Autodesk Fusion 360 part; units mm, degrees
(part 2 of 3)
sketch "Sketch4" plane through (0, 0, 1.5) normal (0, 0, 1) x (-1, 0, 0) in component "Plate"
  line L0 (-48.7193, -101.035) -> (-62.72, -101.035)
  line L1 (-62.72, -101.035) -> (-62.72, -87.0356)
  line L2 (-62.72, -87.0356) -> (-48.7193, -87.0356)
  line L3 (-48.7193, -87.0356) -> (-48.7193, -101.035)
  line L4 (-24.62, -67.9856) -> (-10.6192, -67.9856)
  line L5 (-10.6192, -67.9856) -> (-10.6192, -81.9848)
  line L6 (-10.6192, -81.9848) -> (-24.62, -81.9848)
  line L7 (-24.62, -81.9848) -> (-24.62, -67.9856)
  line L8 (-81.77, -72.4598) -> (-81.77, -58.4606)
  line L9 (-81.77, -58.4606) -> (-77.0696, -58.4606)
  line L10 (-77.0696, -58.4606) -> (-77.0696, -56.9352)
  line L11 (-77.0696, -56.9352) -> (-80.2996, -56.9352)
  line L12 (-80.2996, -56.9352) -> (-80.2996, -55.2097)
  line L13 (-80.2996, -55.2097) -> (-81.219, -55.2097)
  line L14 (-81.219, -55.2097) -> (-81.219, -51.9105)
  line L15 (-81.219, -51.9105) -> (-80.2996, -51.9105)
  line L16 (-80.2996, -51.9105) -> (-80.2996, -50.1855)
  line L17 (-80.2996, -50.1855) -> (-77.0696, -50.1855)
  line L18 (-77.0696, -50.1855) -> (-77.0696, -49.36)
  line L19 (-77.0696, -49.36) -> (-74.2692, -49.36)
  line L20 (-74.2692, -49.36) -> (-74.2692, -50.1855)
  line L21 (-74.2692, -50.1855) -> (-67.9993, -50.1855)
  line L22 (-67.9993, -50.1855) -> (-67.9993, -51.9105)
  line L23 (-67.9993, -51.9105) -> (-67.0197, -51.9105)
  line L24 (-67.0197, -51.9105) -> (-67.0197, -55.2097)
  line L25 (-67.0197, -55.2097) -> (-67.9993, -55.2097)
  line L26 (-67.9993, -55.2097) -> (-67.9993, -56.9352)
  line L27 (-67.9993, -56.9352) -> (-72.4697, -56.9352)
  line L28 (-72.4697, -56.9352) -> (-72.4697, -58.4606)
  line L29 (-72.4697, -58.4606) -> (-67.7693, -58.4606)
  line L30 (-67.7693, -58.4606) -> (-67.7693, -72.4598)
  line L31 (-67.7693, -72.4598) -> (-72.4697, -72.4598)
  line L32 (-72.4697, -72.4598) -> (-72.4697, -73.9856)
  line L33 (-72.4697, -73.9856) -> (-67.9993, -73.9856)
  line L34 (-67.9993, -73.9856) -> (-67.9993, -75.7107)
  line L35 (-67.9993, -75.7107) -> (-67.0197, -75.7107)
  line L36 (-67.0197, -75.7107) -> (-67.0197, -79.0099)
  line L37 (-67.0197, -79.0099) -> (-67.9993, -79.0099)
  line L38 (-67.9993, -79.0099) -> (-67.9993, -80.735)
  line L39 (-67.9993, -80.735) -> (-74.2692, -80.735)
  line L40 (-74.2692, -80.735) -> (-74.2692, -81.5605)
  line L41 (-74.2692, -81.5605) -> (-77.0696, -81.5605)
  line L42 (-77.0696, -81.5605) -> (-77.0696, -80.735)
  line L43 (-77.0696, -80.735) -> (-80.2996, -80.735)
  line L44 (-80.2996, -80.735) -> (-80.2996, -79.0099)
  line L45 (-80.2996, -79.0099) -> (-81.219, -79.0099)
  line L46 (-81.219, -79.0099) -> (-81.219, -75.7107)
  line L47 (-81.219, -75.7107) -> (-80.2996, -75.7107)
  line L48 (-80.2996, -75.7107) -> (-80.2996, -73.9856)
  line L49 (-80.2996, -73.9856) -> (-77.0696, -73.9856)
  line L50 (-77.0696, -73.9856) -> (-77.0696, -72.4598)
  line L51 (-77.0696, -72.4598) -> (-81.77, -72.4598)
  line L52 (-24.62, -101.035) -> (-24.62, -87.0356)
  line L53 (-24.62, -87.0356) -> (-10.6192, -87.0356)
  line L54 (-10.6192, -87.0356) -> (-10.6192, -101.035)
  line L55 (-10.6192, -101.035) -> (-24.62, -101.035)
  line L56 (-31.4446, -129.035) -> (-60.9446, -129.035)
  line L57 (-60.9446, -129.035) -> (-60.9446, -114.035)
  line L58 (-60.9446, -114.035) -> (-31.4446, -114.035)
  line L59 (-31.4446, -114.035) -> (-31.4446, -129.035)
  line L60 (-81.77, -87.0356) -> (-67.7693, -87.0356)
  line L61 (-67.7693, -87.0356) -> (-67.7693, -101.035)
  line L62 (-67.7693, -101.035) -> (-81.77, -101.035)
  line L63 (-81.77, -101.035) -> (-81.77, -87.0356)
  line L64 (-62.72, -67.9856) -> (-48.7193, -67.9856)
  line L65 (-48.7193, -67.9856) -> (-48.7193, -81.9848)
  line L66 (-48.7193, -81.9848) -> (-62.72, -81.9848)
  line L67 (-62.72, -81.9848) -> (-62.72, -67.9856)
  line L68 (-29.6692, -67.9856) -> (-29.6692, -81.9848)
  line L69 (-29.6692, -81.9848) -> (-43.67, -81.9848)
  line L70 (-43.67, -81.9848) -> (-43.67, -67.9856)
  line L71 (-43.67, -67.9856) -> (-29.6692, -67.9856)
  line L72 (-29.6692, -48.9356) -> (-29.6692, -62.9348)
  line L73 (-29.6692, -62.9348) -> (-43.67, -62.9348)
  line L74 (-43.67, -62.9348) -> (-43.67, -48.9356)
  line L75 (-43.67, -48.9356) -> (-29.6692, -48.9356)
  line L76 (-67.9993, -12.0854) -> (-67.9993, -13.8107)
  line L77 (-67.9993, -13.8107) -> (-67.0197, -13.8107)
  line L78 (-67.0197, -13.8107) -> (-67.0197, -17.1097)
  line L79 (-67.0197, -17.1097) -> (-67.9993, -17.1097)
  line L80 (-67.9993, -17.1097) -> (-67.9993, -18.835)
  line L81 (-67.9993, -18.835) -> (-72.4697, -18.835)
  line L82 (-72.4697, -18.835) -> (-72.4697, -20.3605)
  line L83 (-72.4697, -20.3605) -> (-67.7693, -20.3605)
  line L84 (-67.7693, -20.3605) -> (-67.7693, -34.36)
  line L85 (-67.7693, -34.36) -> (-72.4697, -34.36)
  line L86 (-72.4697, -34.36) -> (-72.4697, -35.8856)
  line L87 (-72.4697, -35.8856) -> (-67.9993, -35.8856)
  line L88 (-67.9993, -35.8856) -> (-67.9993, -37.6107)
  line L89 (-67.9993, -37.6107) -> (-67.0197, -37.6107)
  line L90 (-67.0197, -37.6107) -> (-67.0197, -40.9099)
  line L91 (-67.0197, -40.9099) -> (-67.9993, -40.9099)
  line L92 (-67.9993, -40.9099) -> (-67.9993, -42.635)
  line L93 (-67.9993, -42.635) -> (-74.2692, -42.635)
  line L94 (-74.2692, -42.635) -> (-74.2692, -43.4605)
  line L95 (-74.2692, -43.4605) -> (-77.0696, -43.4605)
  line L96 (-77.0696, -43.4605) -> (-77.0696, -42.635)
  line L97 (-77.0696, -42.635) -> (-80.2996, -42.635)
  line L98 (-80.2996, -42.635) -> (-80.2996, -40.9099)
  line L99 (-80.2996, -40.9099) -> (-81.219, -40.9099)
  line L100 (-81.219, -40.9099) -> (-81.219, -37.6107)
  line L101 (-81.219, -37.6107) -> (-80.2996, -37.6107)
  line L102 (-80.2996, -37.6107) -> (-80.2996, -35.8856)
  line L103 (-80.2996, -35.8856) -> (-77.0696, -35.8856)
  line L104 (-77.0696, -35.8856) -> (-77.0696, -34.36)
  line L105 (-77.0696, -34.36) -> (-81.77, -34.36)
  line L106 (-81.77, -34.36) -> (-81.77, -20.3605)
  line L107 (-81.77, -20.3605) -> (-77.0696, -20.3605)
  line L108 (-77.0696, -20.3605) -> (-77.0696, -18.835)
  line L109 (-77.0696, -18.835) -> (-80.2996, -18.835)
  line L110 (-80.2996, -18.835) -> (-80.2996, -17.1097)
  line L111 (-80.2996, -17.1097) -> (-81.219, -17.1097)
  line L112 (-81.219, -17.1097) -> (-81.219, -13.8107)
  line L113 (-81.219, -13.8107) -> (-80.2996, -13.8107)
  line L114 (-80.2996, -13.8107) -> (-80.2996, -12.0854)
  line L115 (-80.2996, -12.0854) -> (-77.0696, -12.0854)
  line L116 (-77.0696, -12.0854) -> (-77.0696, -11.26)
  line L117 (-77.0696, -11.26) -> (-74.2692, -11.26)
  line L118 (-74.2692, -11.26) -> (-74.2692, -12.0854)
  line L119 (-74.2692, -12.0854) -> (-67.9993, -12.0854)
  line L120 (-29.6692, -29.8855) -> (-29.6692, -43.8849)
  line L121 (-29.6692, -43.8849) -> (-43.67, -43.8849)
  line L122 (-43.67, -43.8849) -> (-43.67, -29.8855)
  line L123 (-43.67, -29.8855) -> (-29.6692, -29.8855)
  line L124 (-48.7193, -62.9348) -> (-62.72, -62.9348)
  line L125 (-62.72, -62.9348) -> (-62.72, -48.9356)
  line L126 (-62.72, -48.9356) -> (-48.7193, -48.9356)
  line L127 (-48.7193, -48.9356) -> (-48.7193, -62.9348)
  line L128 (-24.62, -43.8849) -> (-24.62, -29.8855)
  line L129 (-24.62, -29.8855) -> (-10.6192, -29.8855)
  line L130 (-10.6192, -29.8855) -> (-10.6192, -43.8849)
  line L131 (-10.6192, -43.8849) -> (-24.62, -43.8849)
  line L132 (-48.7193, -10.8355) -> (-48.7193, -24.835)
  line L133 (-48.7193, -24.835) -> (-62.72, -24.835)
  line L134 (-62.72, -24.835) -> (-62.72, -10.8355)
  line L135 (-62.72, -10.8355) -> (-48.7193, -10.8355)
  line L136 (-37.3944, -23.3646) -> (-37.3944, -24.2852)
  line L137 (-37.3944, -24.2852) -> (-40.6936, -24.2852)
  line L138 (-40.6936, -24.2852) -> (-40.6936, -23.3646)
  line L139 (-40.6936, -23.3646) -> (-42.4187, -23.3646)
  line L140 (-42.4187, -23.3646) -> (-42.4187, -20.1345)
  line L141 (-42.4187, -20.1345) -> (-43.2442, -20.1345)
  line L142 (-43.2442, -20.1345) -> (-43.2442, -17.3357)
  line L143 (-43.2442, -17.3357) -> (-42.4187, -17.3357)
  line L144 (-42.4187, -17.3357) -> (-42.4187, -11.0657)
  line L145 (-42.4187, -11.0657) -> (-40.6936, -11.0657)
  line L146 (-40.6936, -11.0657) -> (-40.6936, -10.0858)
  line L147 (-40.6936, -10.0858) -> (-37.3944, -10.0858)
  line L148 (-37.3944, -10.0858) -> (-37.3944, -11.0657)
  line L149 (-37.3944, -11.0657) -> (-35.669, -11.0657)
  line L150 (-35.669, -11.0657) -> (-35.669, -15.5346)
  line L151 (-35.669, -15.5346) -> (-34.145, -15.5346)
  line L152 (-34.145, -15.5346) -> (-34.145, -10.8355)
  line L153 (-34.145, -10.8355) -> (-20.1442, -10.8355)
  line L154 (-20.1442, -10.8355) -> (-20.1442, -15.5346)
  line L155 (-20.1442, -15.5346) -> (-18.6201, -15.5346)
  line L156 (-18.6201, -15.5346) -> (-18.6201, -11.0657)
  line L157 (-18.6201, -11.0657) -> (-16.8934, -11.0657)
  line L158 (-16.8934, -11.0657) -> (-16.8934, -10.0858)
  line L159 (-16.8934, -10.0858) -> (-13.593, -10.0858)
  line L160 (-13.593, -10.0858) -> (-13.593, -11.0657)
  line L161 (-13.593, -11.0657) -> (-11.869, -11.0657)
  line L162 (-11.869, -11.0657) -> (-11.869, -17.3357)
  line L163 (-11.869, -17.3357) -> (-11.0436, -17.3357)
  line L164 (-11.0436, -17.3357) -> (-11.0436, -20.1345)
  line L165 (-11.0436, -20.1345) -> (-11.869, -20.1345)
  line L166 (-11.869, -20.1345) -> (-11.869, -23.3646)
  line L167 (-11.869, -23.3646) -> (-13.593, -23.3646)
  line L168 (-13.593, -23.3646) -> (-13.593, -24.2852)
  line L169 (-13.593, -24.2852) -> (-16.8934, -24.2852)
  line L170 (-16.8934, -24.2852) -> (-16.8934, -23.3646)
  line L171 (-16.8934, -23.3646) -> (-18.6201, -23.3646)
  line L172 (-18.6201, -23.3646) -> (-18.6201, -20.1345)
  line L173 (-18.6201, -20.1345) -> (-20.1442, -20.1345)
  line L174 (-20.1442, -20.1345) -> (-20.1442, -24.835)
  line L175 (-20.1442, -24.835) -> (-34.145, -24.835)
  line L176 (-34.145, -24.835) -> (-34.145, -20.1345)
  line L177 (-34.145, -20.1345) -> (-35.669, -20.1345)
  line L178 (-35.669, -20.1345) -> (-35.669, -23.3646)
  line L179 (-35.669, -23.3646) -> (-37.3944, -23.3646)
  line L180 (-62.72, -43.8849) -> (-62.72, -29.8855)
  line L181 (-62.72, -29.8855) -> (-48.7193, -29.8855)
  line L182 (-48.7193, -29.8855) -> (-48.7193, -43.8849)
  line L183 (-48.7193, -43.8849) -> (-62.72, -43.8849)
  line L184 (-43.67, -87.0356) -> (-29.6692, -87.0356)
  line L185 (-29.6692, -87.0356) -> (-29.6692, -101.035)
  line L186 (-29.6692, -101.035) -> (-43.67, -101.035)
  line L187 (-43.67, -101.035) -> (-43.67, -87.0356)
  line L188 (-24.62, -62.9348) -> (-24.62, -48.9356)
  line L189 (-24.62, -48.9356) -> (-10.6192, -48.9356)
  line L190 (-10.6192, -48.9356) -> (-10.6192, -62.9348)
  line L191 (-10.6192, -62.9348) -> (-24.62, -62.9348)
  arc A0 (-6.6192, -142.035) -> (-4.6192, -140.035) centre (-6.6192, -140.035) ccw
  line L192 (-4.6192, -140.035) -> (-4.6192, -6.8355)
  arc A1 (-4.6192, -6.8355) -> (-6.6192, -4.8355) centre (-6.6192, -6.8355) ccw
  line L193 (-6.6192, -4.8355) -> (-85.77, -4.8355)
  arc A2 (-85.77, -4.8355) -> (-87.77, -6.8355) centre (-85.77, -6.8355) ccw
  line L194 (-87.77, -6.8355) -> (-87.77, -140.035)
  arc A3 (-87.77, -140.035) -> (-85.77, -142.035) centre (-85.77, -140.035) ccw
  line L195 (-85.77, -142.035) -> (-6.6192, -142.035)
  line L196 (-31.4446, -129.035) -> (-60.9446, -129.035)
  line L197 (-31.4446, -114.035) -> (-31.4446, -129.035)
  line L198 (-60.9446, -114.035) -> (-31.4446, -114.035)
  line L199 (-60.9446, -129.035) -> (-60.9446, -114.035)
  line L200 (-10.6192, -114.5353) -> (-10.6192, -128.5347)
  line L201 (-10.6192, -128.5347) -> (-24.62, -128.5347)
  line L202 (-24.62, -128.5347) -> (-24.62, -114.5353)
  line L203 (-24.62, -114.5353) -> (-10.6192, -114.5353)
sketch "Sketch5" plane through (0, 0, 0) normal (0, 0, -1) x (1, 0, 0) in component "Plate"
  line L0 (62.72, -101.035) -> (48.7193, -101.035)
  line L1 (48.7193, -101.035) -> (48.7193, -87.0356)
  line L2 (48.7193, -87.0356) -> (62.72, -87.0356)
  line L3 (62.72, -87.0356) -> (62.72, -101.035)
  line L4 (10.6192, -67.9856) -> (24.62, -67.9856)
  line L5 (24.62, -67.9856) -> (24.62, -81.9848)
  line L6 (24.62, -81.9848) -> (10.6192, -81.9848)
  line L7 (10.6192, -81.9848) -> (10.6192, -67.9856)
  line L8 (81.77, -58.4606) -> (81.77, -72.4598)
  line L9 (81.77, -72.4598) -> (77.0696, -72.4598)
  line L10 (77.0696, -72.4598) -> (77.0696, -73.9856)
  line L11 (77.0696, -73.9856) -> (80.2996, -73.9856)
  line L12 (80.2996, -73.9856) -> (80.2996, -75.7107)
  line L13 (80.2996, -75.7107) -> (81.219, -75.7107)
  line L14 (81.219, -75.7107) -> (81.219, -79.0099)
  line L15 (81.219, -79.0099) -> (80.2996, -79.0099)
  line L16 (80.2996, -79.0099) -> (80.2996, -80.735)
  line L17 (80.2996, -80.735) -> (77.0696, -80.735)
  line L18 (77.0696, -80.735) -> (77.0696, -81.5605)
  line L19 (77.0696, -81.5605) -> (74.2692, -81.5605)
  line L20 (74.2692, -81.5605) -> (74.2692, -80.735)
  line L21 (74.2692, -80.735) -> (67.9993, -80.735)
  line L22 (67.9993, -80.735) -> (67.9993, -79.0099)
  line L23 (67.9993, -79.0099) -> (67.0197, -79.0099)
  line L24 (67.0197, -79.0099) -> (67.0197, -75.7107)
  line L25 (67.0197, -75.7107) -> (67.9993, -75.7107)
  line L26 (67.9993, -75.7107) -> (67.9993, -73.9856)
  line L27 (67.9993, -73.9856) -> (72.4697, -73.9856)
  line L28 (72.4697, -73.9856) -> (72.4697, -72.4598)
  line L29 (72.4697, -72.4598) -> (67.7693, -72.4598)
  line L30 (67.7693, -72.4598) -> (67.7693, -58.4606)
  line L31 (67.7693, -58.4606) -> (72.4697, -58.4606)
  line L32 (72.4697, -58.4606) -> (72.4697, -56.9352)
  line L33 (72.4697, -56.9352) -> (67.9993, -56.9352)
  line L34 (67.9993, -56.9352) -> (67.9993, -55.2097)
  line L35 (67.9993, -55.2097) -> (67.0197, -55.2097)
  line L36 (67.0197, -55.2097) -> (67.0197, -51.9105)
  line L37 (67.0197, -51.9105) -> (67.9993, -51.9105)
  line L38 (67.9993, -51.9105) -> (67.9993, -50.1855)
  line L39 (67.9993, -50.1855) -> (74.2692, -50.1855)
  line L40 (74.2692, -50.1855) -> (74.2692, -49.36)
  line L41 (74.2692, -49.36) -> (77.0696, -49.36)
  line L42 (77.0696, -49.36) -> (77.0696, -50.1855)
  line L43 (77.0696, -50.1855) -> (80.2996, -50.1855)
  line L44 (80.2996, -50.1855) -> (80.2996, -51.9105)
  line L45 (80.2996, -51.9105) -> (81.219, -51.9105)
  line L46 (81.219, -51.9105) -> (81.219, -55.2097)
  line L47 (81.219, -55.2097) -> (80.2996, -55.2097)
  line L48 (80.2996, -55.2097) -> (80.2996, -56.9352)
  line L49 (80.2996, -56.9352) -> (77.0696, -56.9352)
  line L50 (77.0696, -56.9352) -> (77.0696, -58.4606)
  line L51 (77.0696, -58.4606) -> (81.77, -58.4606)
  line L52 (24.62, -87.0356) -> (24.62, -101.035)
  line L53 (24.62, -101.035) -> (10.6192, -101.035)
  line L54 (10.6192, -101.035) -> (10.6192, -87.0356)
  line L55 (10.6192, -87.0356) -> (24.62, -87.0356)
  line L56 (60.9446, -129.035) -> (31.4446, -129.035)
  line L57 (31.4446, -129.035) -> (31.4446, -114.035)
  line L58 (31.4446, -114.035) -> (60.9446, -114.035)
  line L59 (60.9446, -114.035) -> (60.9446, -129.035)
  line L60 (67.7693, -87.0356) -> (81.77, -87.0356)
  line L61 (81.77, -87.0356) -> (81.77, -101.035)
  line L62 (81.77, -101.035) -> (67.7693, -101.035)
  line L63 (67.7693, -101.035) -> (67.7693, -87.0356)
  line L64 (48.7193, -67.9856) -> (62.72, -67.9856)
  line L65 (62.72, -67.9856) -> (62.72, -81.9848)
  line L66 (62.72, -81.9848) -> (48.7193, -81.9848)
  line L67 (48.7193, -81.9848) -> (48.7193, -67.9856)
  line L68 (29.6692, -81.9848) -> (29.6692, -67.9856)
  line L69 (29.6692, -67.9856) -> (43.67, -67.9856)
  line L70 (43.67, -67.9856) -> (43.67, -81.9848)
  line L71 (43.67, -81.9848) -> (29.6692, -81.9848)
  line L72 (29.6692, -62.9348) -> (29.6692, -48.9356)
  line L73 (29.6692, -48.9356) -> (43.67, -48.9356)
  line L74 (43.67, -48.9356) -> (43.67, -62.9348)
  line L75 (43.67, -62.9348) -> (29.6692, -62.9348)
  line L76 (67.9993, -13.8107) -> (67.9993, -12.0854)
  line L77 (67.9993, -12.0854) -> (74.2692, -12.0854)
  line L78 (74.2692, -12.0854) -> (74.2692, -11.26)
  line L79 (74.2692, -11.26) -> (77.0696, -11.26)
  line L80 (77.0696, -11.26) -> (77.0696, -12.0854)
  line L81 (77.0696, -12.0854) -> (80.2996, -12.0854)
  line L82 (80.2996, -12.0854) -> (80.2996, -13.8107)
  line L83 (80.2996, -13.8107) -> (81.219, -13.8107)
  line L84 (81.219, -13.8107) -> (81.219, -17.1097)
  line L85 (81.219, -17.1097) -> (80.2996, -17.1097)
  line L86 (80.2996, -17.1097) -> (80.2996, -18.835)
  line L87 (80.2996, -18.835) -> (77.0696, -18.835)
  line L88 (77.0696, -18.835) -> (77.0696, -20.3605)
  line L89 (77.0696, -20.3605) -> (81.77, -20.3605)
  line L90 (81.77, -20.3605) -> (81.77, -34.36)
  line L91 (81.77, -34.36) -> (77.0696, -34.36)
  line L92 (77.0696, -34.36) -> (77.0696, -35.8856)
  line L93 (77.0696, -35.8856) -> (80.2996, -35.8856)
  line L94 (80.2996, -35.8856) -> (80.2996, -37.6107)
  line L95 (80.2996, -37.6107) -> (81.219, -37.6107)
  line L96 (81.219, -37.6107) -> (81.219, -40.9099)
  line L97 (81.219, -40.9099) -> (80.2996, -40.9099)
  line L98 (80.2996, -40.9099) -> (80.2996, -42.635)
  line L99 (80.2996, -42.635) -> (77.0696, -42.635)
  line L100 (77.0696, -42.635) -> (77.0696, -43.4605)
  line L101 (77.0696, -43.4605) -> (74.2692, -43.4605)
  line L102 (74.2692, -43.4605) -> (74.2692, -42.635)
  line L103 (74.2692, -42.635) -> (67.9993, -42.635)
  line L104 (67.9993, -42.635) -> (67.9993, -40.9099)
  line L105 (67.9993, -40.9099) -> (67.0197, -40.9099)
  line L106 (67.0197, -40.9099) -> (67.0197, -37.6107)
  line L107 (67.0197, -37.6107) -> (67.9993, -37.6107)
  line L108 (67.9993, -37.6107) -> (67.9993, -35.8856)
  line L109 (67.9993, -35.8856) -> (72.4697, -35.8856)
  line L110 (72.4697, -35.8856) -> (72.4697, -34.36)
  line L111 (72.4697, -34.36) -> (67.7693, -34.36)
  line L112 (67.7693, -34.36) -> (67.7693, -20.3605)
  line L113 (67.7693, -20.3605) -> (72.4697, -20.3605)
  line L114 (72.4697, -20.3605) -> (72.4697, -18.835)
  line L115 (72.4697, -18.835) -> (67.9993, -18.835)
  line L116 (67.9993, -18.835) -> (67.9993, -17.1097)
  line L117 (67.9993, -17.1097) -> (67.0197, -17.1097)
  line L118 (67.0197, -17.1097) -> (67.0197, -13.8107)
  line L119 (67.0197, -13.8107) -> (67.9993, -13.8107)
  line L120 (29.6692, -43.8849) -> (29.6692, -29.8855)
  line L121 (29.6692, -29.8855) -> (43.67, -29.8855)
  line L122 (43.67, -29.8855) -> (43.67, -43.8849)
  line L123 (43.67, -43.8849) -> (29.6692, -43.8849)
  line L124 (62.72, -62.9348) -> (48.7193, -62.9348)
  line L125 (48.7193, -62.9348) -> (48.7193, -48.9356)
  line L126 (48.7193, -48.9356) -> (62.72, -48.9356)
  line L127 (62.72, -48.9356) -> (62.72, -62.9348)
  line L128 (24.62, -29.8855) -> (24.62, -43.8849)
  line L129 (24.62, -43.8849) -> (10.6192, -43.8849)
  line L130 (10.6192, -43.8849) -> (10.6192, -29.8855)
  line L131 (10.6192, -29.8855) -> (24.62, -29.8855)
  line L132 (48.7193, -24.835) -> (48.7193, -10.8355)
  line L133 (48.7193, -10.8355) -> (62.72, -10.8355)
  line L134 (62.72, -10.8355) -> (62.72, -24.835)
  line L135 (62.72, -24.835) -> (48.7193, -24.835)
  line L136 (37.3944, -24.2852) -> (37.3944, -23.3646)
  line L137 (37.3944, -23.3646) -> (35.669, -23.3646)
  line L138 (35.669, -23.3646) -> (35.669, -20.1345)
  line L139 (35.669, -20.1345) -> (34.145, -20.1345)
  line L140 (34.145, -20.1345) -> (34.145, -24.835)
  line L141 (34.145, -24.835) -> (20.1442, -24.835)
  line L142 (20.1442, -24.835) -> (20.1442, -20.1345)
  line L143 (20.1442, -20.1345) -> (18.6201, -20.1345)
  line L144 (18.6201, -20.1345) -> (18.6201, -23.3646)
  line L145 (18.6201, -23.3646) -> (16.8934, -23.3646)
  line L146 (16.8934, -23.3646) -> (16.8934, -24.2852)
  line L147 (16.8934, -24.2852) -> (13.593, -24.2852)
  line L148 (13.593, -24.2852) -> (13.593, -23.3646)
  line L149 (13.593, -23.3646) -> (11.869, -23.3646)
  line L150 (11.869, -23.3646) -> (11.869, -20.1345)
  line L151 (11.869, -20.1345) -> (11.0436, -20.1345)
  line L152 (11.0436, -20.1345) -> (11.0436, -17.3357)
  line L153 (11.0436, -17.3357) -> (11.869, -17.3357)
  line L154 (11.869, -17.3357) -> (11.869, -11.0657)
  line L155 (11.869, -11.0657) -> (13.593, -11.0657)
  line L156 (13.593, -11.0657) -> (13.593, -10.0858)
  line L157 (13.593, -10.0858) -> (16.8934, -10.0858)
  line L158 (16.8934, -10.0858) -> (16.8934, -11.0657)
  line L159 (16.8934, -11.0657) -> (18.6201, -11.0657)
  line L160 (18.6201, -11.0657) -> (18.6201, -15.5346)
  line L161 (18.6201, -15.5346) -> (20.1442, -15.5346)
  line L162 (20.1442, -15.5346) -> (20.1442, -10.8355)
  line L163 (20.1442, -10.8355) -> (34.145, -10.8355)
  line L164 (34.145, -10.8355) -> (34.145, -15.5346)
  line L165 (34.145, -15.5346) -> (35.669, -15.5346)
  line L166 (35.669, -15.5346) -> (35.669, -11.0657)
  line L167 (35.669, -11.0657) -> (37.3944, -11.0657)
  line L168 (37.3944, -11.0657) -> (37.3944, -10.0858)
  line L169 (37.3944, -10.0858) -> (40.6936, -10.0858)
  line L170 (40.6936, -10.0858) -> (40.6936, -11.0657)
  line L171 (40.6936, -11.0657) -> (42.4187, -11.0657)
  line L172 (42.4187, -11.0657) -> (42.4187, -17.3357)
  line L173 (42.4187, -17.3357) -> (43.2442, -17.3357)
  line L174 (43.2442, -17.3357) -> (43.2442, -20.1345)
  line L175 (43.2442, -20.1345) -> (42.4187, -20.1345)
  line L176 (42.4187, -20.1345) -> (42.4187, -23.3646)
  line L177 (42.4187, -23.3646) -> (40.6936, -23.3646)
  line L178 (40.6936, -23.3646) -> (40.6936, -24.2852)
  line L179 (40.6936, -24.2852) -> (37.3944, -24.2852)
  line L180 (62.72, -29.8855) -> (62.72, -43.8849)
  line L181 (62.72, -43.8849) -> (48.7193, -43.8849)
  line L182 (48.7193, -43.8849) -> (48.7193, -29.8855)
  line L183 (48.7193, -29.8855) -> (62.72, -29.8855)
  line L184 (29.6692, -87.0356) -> (43.67, -87.0356)
  line L185 (43.67, -87.0356) -> (43.67, -101.035)
  line L186 (43.67, -101.035) -> (29.6692, -101.035)
  line L187 (29.6692, -101.035) -> (29.6692, -87.0356)
  line L188 (24.62, -48.9356) -> (24.62, -62.9348)
  line L189 (24.62, -62.9348) -> (10.6192, -62.9348)
  line L190 (10.6192, -62.9348) -> (10.6192, -48.9356)
  line L191 (10.6192, -48.9356) -> (24.62, -48.9356)
  arc A0 (4.6192, -140.035) -> (6.6192, -142.035) centre (6.6192, -140.035) ccw
  line L192 (6.6192, -142.035) -> (85.77, -142.035)
  arc A1 (85.77, -142.035) -> (87.77, -140.035) centre (85.77, -140.035) ccw
  line L193 (87.77, -140.035) -> (87.77, -6.8355)
  arc A2 (87.77, -6.8355) -> (85.77, -4.8355) centre (85.77, -6.8355) ccw
  line L194 (85.77, -4.8355) -> (6.6192, -4.8355)
  arc A3 (6.6192, -4.8355) -> (4.6192, -6.8355) centre (6.6192, -6.8355) ccw
  line L195 (4.6192, -6.8355) -> (4.6192, -140.035)
  circle A4 centre (7.6799, -138.9743) radius 1
  line L196 (10.6192, -128.5347) -> (10.6192, -114.5353)
  line L197 (10.6192, -114.5353) -> (24.62, -114.5353)
  line L198 (24.62, -114.5353) -> (24.62, -128.5347)
  line L199 (24.62, -128.5347) -> (10.6192, -128.5347)
  line L200 (5.205, -141.4492) -> (7.6799, -138.9743) construction
  line L201 (5.205, -141.4492) -> (8.705, -141.4492) construction
  dimension "d122" = 2
  dimension "d188" = 45
  dimension "d189" = 3.5
  constraint horizontal L201
  constraint midpoint A0 L200.start
  constraint coincident A4.centre L200.end
  measures "d122" diameter of A4
  measures "d188" angle of L200 L201
  measures "d189" distance of L200.start A4.centre
ref_plane "WorkPlane1" through (46.1946, 73.4353, 4.9) normal (0, 0, 1) x (1, 0, 0) in component "Plate"
extrude "Extrude2'" cut sketch "Sketch5" against normal up to surface (4.9 mm away) contours A4 bodies 1 in component "Plate"
extrude "Extrude6" cut sketch "Sketch5" against normal up to surface (4.9 mm away) contours A4 bodies 2 in component "Top"
ref_plane "WorkPlane1" through (46.1946, 73.4353, 1.075) normal (-1, 0, 0) x (0, 0, 1) in component "Top"
ref_plane "WorkPlane2" through (46.1946, 73.4353, 1.075) normal (0, 1, 0) x (0, 0, 1) in component "Top"
mirror "Mirror1" about plane through (46.1946, 73.4353, 1.075) normal (-1, 0, 0) of "Extrude2'" in component "Plate"
mirror "Mirror1'" about plane through (46.1946, 73.4353, 1.075) normal (-1, 0, 0) of "Extrude6" in component "Top"
sketch "Sketch6" plane through (0, 0, 0) normal (0, 0, -1) x (1, 0, 0) in component "Plate"
  circle A0 centre (84.7093, -138.9743) radius 1
  circle A1 centre (7.6799, -138.9743) radius 1
  line L0 (62.72, -101.035) -> (48.7193, -101.035)
  line L1 (48.7193, -101.035) -> (48.7193, -87.0356)
  line L2 (48.7193, -87.0356) -> (62.72, -87.0356)
  line L3 (62.72, -87.0356) -> (62.72, -101.035)
  line L4 (10.6192, -67.9856) -> (24.62, -67.9856)
  line L5 (24.62, -67.9856) -> (24.62, -81.9848)
  line L6 (24.62, -81.9848) -> (10.6192, -81.9848)
  line L7 (10.6192, -81.9848) -> (10.6192, -67.9856)
  line L8 (81.77, -58.4606) -> (81.77, -72.4598)
  line L9 (81.77, -72.4598) -> (77.0696, -72.4598)
  line L10 (77.0696, -72.4598) -> (77.0696, -73.9856)
  line L11 (77.0696, -73.9856) -> (80.2996, -73.9856)
  line L12 (80.2996, -73.9856) -> (80.2996, -75.7107)
  line L13 (80.2996, -75.7107) -> (81.219, -75.7107)
  line L14 (81.219, -75.7107) -> (81.219, -79.0099)
  line L15 (81.219, -79.0099) -> (80.2996, -79.0099)
  line L16 (80.2996, -79.0099) -> (80.2996, -80.735)
  line L17 (80.2996, -80.735) -> (77.0696, -80.735)
  line L18 (77.0696, -80.735) -> (77.0696, -81.5605)
  line L19 (77.0696, -81.5605) -> (74.2692, -81.5605)
  line L20 (74.2692, -81.5605) -> (74.2692, -80.735)
  line L21 (74.2692, -80.735) -> (67.9993, -80.735)
  line L22 (67.9993, -80.735) -> (67.9993, -79.0099)
  line L23 (67.9993, -79.0099) -> (67.0197, -79.0099)
  line L24 (67.0197, -79.0099) -> (67.0197, -75.7107)
  line L25 (67.0197, -75.7107) -> (67.9993, -75.7107)
  line L26 (67.9993, -75.7107) -> (67.9993, -73.9856)
  line L27 (67.9993, -73.9856) -> (72.4697, -73.9856)
  line L28 (72.4697, -73.9856) -> (72.4697, -72.4598)
  line L29 (72.4697, -72.4598) -> (67.7693, -72.4598)
  line L30 (67.7693, -72.4598) -> (67.7693, -58.4606)
  line L31 (67.7693, -58.4606) -> (72.4697, -58.4606)
  line L32 (72.4697, -58.4606) -> (72.4697, -56.9352)
  line L33 (72.4697, -56.9352) -> (67.9993, -56.9352)
  line L34 (67.9993, -56.9352) -> (67.9993, -55.2097)
  line L35 (67.9993, -55.2097) -> (67.0197, -55.2097)
  line L36 (67.0197, -55.2097) -> (67.0197, -51.9105)
  line L37 (67.0197, -51.9105) -> (67.9993, -51.9105)
  line L38 (67.9993, -51.9105) -> (67.9993, -50.1855)
  line L39 (67.9993, -50.1855) -> (74.2692, -50.1855)
  line L40 (74.2692, -50.1855) -> (74.2692, -49.36)
  line L41 (74.2692, -49.36) -> (77.0696, -49.36)
  line L42 (77.0696, -49.36) -> (77.0696, -50.1855)
  line L43 (77.0696, -50.1855) -> (80.2996, -50.1855)
  line L44 (80.2996, -50.1855) -> (80.2996, -51.9105)
  line L45 (80.2996, -51.9105) -> (81.219, -51.9105)
  line L46 (81.219, -51.9105) -> (81.219, -55.2097)
  line L47 (81.219, -55.2097) -> (80.2996, -55.2097)
  line L48 (80.2996, -55.2097) -> (80.2996, -56.9352)
  line L49 (80.2996, -56.9352) -> (77.0696, -56.9352)
  line L50 (77.0696, -56.9352) -> (77.0696, -58.4606)
  line L51 (77.0696, -58.4606) -> (81.77, -58.4606)
  line L52 (24.62, -87.0356) -> (24.62, -101.035)
  line L53 (24.62, -101.035) -> (10.6192, -101.035)
  line L54 (10.6192, -101.035) -> (10.6192, -87.0356)
  line L55 (10.6192, -87.0356) -> (24.62, -87.0356)
  line L56 (60.9446, -129.035) -> (31.4446, -129.035)
  line L57 (31.4446, -129.035) -> (31.4446, -114.035)
  line L58 (31.4446, -114.035) -> (60.9446, -114.035)
  line L59 (60.9446, -114.035) -> (60.9446, -129.035)
  line L60 (67.7693, -87.0356) -> (81.77, -87.0356)
  line L61 (81.77, -87.0356) -> (81.77, -101.035)
  line L62 (81.77, -101.035) -> (67.7693, -101.035)
  line L63 (67.7693, -101.035) -> (67.7693, -87.0356)
  line L64 (48.7193, -67.9856) -> (62.72, -67.9856)
  line L65 (62.72, -67.9856) -> (62.72, -81.9848)
  line L66 (62.72, -81.9848) -> (48.7193, -81.9848)
  line L67 (48.7193, -81.9848) -> (48.7193, -67.9856)
  line L68 (29.6692, -81.9848) -> (29.6692, -67.9856)
  line L69 (29.6692, -67.9856) -> (43.67, -67.9856)
  line L70 (43.67, -67.9856) -> (43.67, -81.9848)
  line L71 (43.67, -81.9848) -> (29.6692, -81.9848)
  line L72 (29.6692, -62.9348) -> (29.6692, -48.9356)
  line L73 (29.6692, -48.9356) -> (43.67, -48.9356)
  line L74 (43.67, -48.9356) -> (43.67, -62.9348)
  line L75 (43.67, -62.9348) -> (29.6692, -62.9348)
  line L76 (67.9993, -13.8107) -> (67.9993, -12.0854)
  line L77 (67.9993, -12.0854) -> (74.2692, -12.0854)
  line L78 (74.2692, -12.0854) -> (74.2692, -11.26)
  line L79 (74.2692, -11.26) -> (77.0696, -11.26)
  line L80 (77.0696, -11.26) -> (77.0696, -12.0854)
  line L81 (77.0696, -12.0854) -> (80.2996, -12.0854)
  line L82 (80.2996, -12.0854) -> (80.2996, -13.8107)
  line L83 (80.2996, -13.8107) -> (81.219, -13.8107)
  line L84 (81.219, -13.8107) -> (81.219, -17.1097)
  line L85 (81.219, -17.1097) -> (80.2996, -17.1097)
  line L86 (80.2996, -17.1097) -> (80.2996, -18.835)
  line L87 (80.2996, -18.835) -> (77.0696, -18.835)
  line L88 (77.0696, -18.835) -> (77.0696, -20.3605)
  line L89 (77.0696, -20.3605) -> (81.77, -20.3605)
  line L90 (81.77, -20.3605) -> (81.77, -34.36)
  line L91 (81.77, -34.36) -> (77.0696, -34.36)
  line L92 (77.0696, -34.36) -> (77.0696, -35.8856)
  line L93 (77.0696, -35.8856) -> (80.2996, -35.8856)
  line L94 (80.2996, -35.8856) -> (80.2996, -37.6107)
  line L95 (80.2996, -37.6107) -> (81.219, -37.6107)
  line L96 (81.219, -37.6107) -> (81.219, -40.9099)
  line L97 (81.219, -40.9099) -> (80.2996, -40.9099)
  line L98 (80.2996, -40.9099) -> (80.2996, -42.635)
  line L99 (80.2996, -42.635) -> (77.0696, -42.635)
  line L100 (77.0696, -42.635) -> (77.0696, -43.4605)
  line L101 (77.0696, -43.4605) -> (74.2692, -43.4605)
  line L102 (74.2692, -43.4605) -> (74.2692, -42.635)
  line L103 (74.2692, -42.635) -> (67.9993, -42.635)
  line L104 (67.9993, -42.635) -> (67.9993, -40.9099)
  line L105 (67.9993, -40.9099) -> (67.0197, -40.9099)
  line L106 (67.0197, -40.9099) -> (67.0197, -37.6107)
  line L107 (67.0197, -37.6107) -> (67.9993, -37.6107)
  line L108 (67.9993, -37.6107) -> (67.9993, -35.8856)
  line L109 (67.9993, -35.8856) -> (72.4697, -35.8856)
  line L110 (72.4697, -35.8856) -> (72.4697, -34.36)
  line L111 (72.4697, -34.36) -> (67.7693, -34.36)
  line L112 (67.7693, -34.36) -> (67.7693, -20.3605)
  line L113 (67.7693, -20.3605) -> (72.4697, -20.3605)
  line L114 (72.4697, -20.3605) -> (72.4697, -18.835)
  line L115 (72.4697, -18.835) -> (67.9993, -18.835)
  line L116 (67.9993, -18.835) -> (67.9993, -17.1097)
  line L117 (67.9993, -17.1097) -> (67.0197, -17.1097)
  line L118 (67.0197, -17.1097) -> (67.0197, -13.8107)
  line L119 (67.0197, -13.8107) -> (67.9993, -13.8107)
  line L120 (29.6692, -43.8849) -> (29.6692, -29.8855)
  line L121 (29.6692, -29.8855) -> (43.67, -29.8855)
  line L122 (43.67, -29.8855) -> (43.67, -43.8849)
  line L123 (43.67, -43.8849) -> (29.6692, -43.8849)
  line L124 (62.72, -62.9348) -> (48.7193, -62.9348)
  line L125 (48.7193, -62.9348) -> (48.7193, -48.9356)
  line L126 (48.7193, -48.9356) -> (62.72, -48.9356)
  line L127 (62.72, -48.9356) -> (62.72, -62.9348)
  line L128 (24.62, -29.8855) -> (24.62, -43.8849)
  line L129 (24.62, -43.8849) -> (10.6192, -43.8849)
  line L130 (10.6192, -43.8849) -> (10.6192, -29.8855)
  line L131 (10.6192, -29.8855) -> (24.62, -29.8855)
  line L132 (48.7193, -24.835) -> (48.7193, -10.8355)
  line L133 (48.7193, -10.8355) -> (62.72, -10.8355)
  line L134 (62.72, -10.8355) -> (62.72, -24.835)
  line L135 (62.72, -24.835) -> (48.7193, -24.835)
  line L136 (37.3944, -24.2852) -> (37.3944, -23.3646)
  line L137 (37.3944, -23.3646) -> (35.669, -23.3646)
  line L138 (35.669, -23.3646) -> (35.669, -20.1345)
  line L139 (35.669, -20.1345) -> (34.145, -20.1345)
  line L140 (34.145, -20.1345) -> (34.145, -24.835)
  line L141 (34.145, -24.835) -> (20.1442, -24.835)
  line L142 (20.1442, -24.835) -> (20.1442, -20.1345)
  line L143 (20.1442, -20.1345) -> (18.6201, -20.1345)
  line L144 (18.6201, -20.1345) -> (18.6201, -23.3646)
  line L145 (18.6201, -23.3646) -> (16.8934, -23.3646)
  line L146 (16.8934, -23.3646) -> (16.8934, -24.2852)
  line L147 (16.8934, -24.2852) -> (13.593, -24.2852)
  line L148 (13.593, -24.2852) -> (13.593, -23.3646)
  line L149 (13.593, -23.3646) -> (11.869, -23.3646)
  line L150 (11.869, -23.3646) -> (11.869, -20.1345)
  line L151 (11.869, -20.1345) -> (11.0436, -20.1345)
  line L152 (11.0436, -20.1345) -> (11.0436, -17.3357)
  line L153 (11.0436, -17.3357) -> (11.869, -17.3357)
  line L154 (11.869, -17.3357) -> (11.869, -11.0657)
  line L155 (11.869, -11.0657) -> (13.593, -11.0657)
  line L156 (13.593, -11.0657) -> (13.593, -10.0858)
  line L157 (13.593, -10.0858) -> (16.8934, -10.0858)
  line L158 (16.8934, -10.0858) -> (16.8934, -11.0657)
  line L159 (16.8934, -11.0657) -> (18.6201, -11.0657)
  line L160 (18.6201, -11.0657) -> (18.6201, -15.5346)
  line L161 (18.6201, -15.5346) -> (20.1442, -15.5346)
  line L162 (20.1442, -15.5346) -> (20.1442, -10.8355)
  line L163 (20.1442, -10.8355) -> (34.145, -10.8355)
  line L164 (34.145, -10.8355) -> (34.145, -15.5346)
  line L165 (34.145, -15.5346) -> (35.669, -15.5346)
  line L166 (35.669, -15.5346) -> (35.669, -11.0657)
  line L167 (35.669, -11.0657) -> (37.3944, -11.0657)
  line L168 (37.3944, -11.0657) -> (37.3944, -10.0858)
  line L169 (37.3944, -10.0858) -> (40.6936, -10.0858)
  line L170 (40.6936, -10.0858) -> (40.6936, -11.0657)
  line L171 (40.6936, -11.0657) -> (42.4187, -11.0657)
  line L172 (42.4187, -11.0657) -> (42.4187, -17.3357)
  line L173 (42.4187, -17.3357) -> (43.2442, -17.3357)
  line L174 (43.2442, -17.3357) -> (43.2442, -20.1345)
  line L175 (43.2442, -20.1345) -> (42.4187, -20.1345)
  line L176 (42.4187, -20.1345) -> (42.4187, -23.3646)
  line L177 (42.4187, -23.3646) -> (40.6936, -23.3646)
  line L178 (40.6936, -23.3646) -> (40.6936, -24.2852)
  line L179 (40.6936, -24.2852) -> (37.3944, -24.2852)
  line L180 (62.72, -29.8855) -> (62.72, -43.8849)
  line L181 (62.72, -43.8849) -> (48.7193, -43.8849)
  line L182 (48.7193, -43.8849) -> (48.7193, -29.8855)
  line L183 (48.7193, -29.8855) -> (62.72, -29.8855)
  line L184 (29.6692, -87.0356) -> (43.67, -87.0356)
  line L185 (43.67, -87.0356) -> (43.67, -101.035)
  line L186 (43.67, -101.035) -> (29.6692, -101.035)
  line L187 (29.6692, -101.035) -> (29.6692, -87.0356)
  line L188 (24.62, -48.9356) -> (24.62, -62.9348)
  line L189 (24.62, -62.9348) -> (10.6192, -62.9348)
  line L190 (10.6192, -62.9348) -> (10.6192, -48.9356)
  line L191 (10.6192, -48.9356) -> (24.62, -48.9356)
  arc A2 (4.6192, -140.035) -> (6.6192, -142.035) centre (6.6192, -140.035) ccw
  line L192 (6.6192, -142.035) -> (85.77, -142.035)
  arc A3 (85.77, -142.035) -> (87.77, -140.035) centre (85.77, -140.035) ccw
  line L193 (87.77, -140.035) -> (87.77, -6.8355)
  arc A4 (87.77, -6.8355) -> (85.77, -4.8355) centre (85.77, -6.8355) ccw
  line L194 (85.77, -4.8355) -> (6.6192, -4.8355)
  arc A5 (6.6192, -4.8355) -> (4.6192, -6.8355) centre (6.6192, -6.8355) ccw
  line L195 (4.6192, -6.8355) -> (4.6192, -140.035)
  line L196 (10.6192, -128.5347) -> (10.6192, -114.5353)
  line L197 (10.6192, -114.5353) -> (24.62, -114.5353)
  line L198 (24.62, -114.5353) -> (24.62, -128.5347)
  line L199 (24.62, -128.5347) -> (10.6192, -128.5347)
sketch "Sketch7" plane through (0, 0, 0) normal (0, 0, -1) x (1, 0, 0) in component "Plate"
  circle A0 centre (84.7093, -138.9743) radius 1
  circle A1 centre (7.6799, -138.9743) radius 1
  line L0 (62.72, -101.035) -> (48.7193, -101.035)
  line L1 (48.7193, -101.035) -> (48.7193, -87.0356)
  line L2 (48.7193, -87.0356) -> (62.72, -87.0356)
  line L3 (62.72, -87.0356) -> (62.72, -101.035)
  line L4 (10.6192, -67.9856) -> (24.62, -67.9856)
  line L5 (24.62, -67.9856) -> (24.62, -81.9848)
  line L6 (24.62, -81.9848) -> (10.6192, -81.9848)
  line L7 (10.6192, -81.9848) -> (10.6192, -67.9856)
  line L8 (81.77, -58.4606) -> (81.77, -72.4598)
  line L9 (81.77, -72.4598) -> (77.0696, -72.4598)
  line L10 (77.0696, -72.4598) -> (77.0696, -73.9856)
  line L11 (77.0696, -73.9856) -> (80.2996, -73.9856)
  line L12 (80.2996, -73.9856) -> (80.2996, -75.7107)
  line L13 (80.2996, -75.7107) -> (81.219, -75.7107)
  line L14 (81.219, -75.7107) -> (81.219, -79.0099)
  line L15 (81.219, -79.0099) -> (80.2996, -79.0099)
  line L16 (80.2996, -79.0099) -> (80.2996, -80.735)
  line L17 (80.2996, -80.735) -> (77.0696, -80.735)
  line L18 (77.0696, -80.735) -> (77.0696, -81.5605)
  line L19 (77.0696, -81.5605) -> (74.2692, -81.5605)
  line L20 (74.2692, -81.5605) -> (74.2692, -80.735)
  line L21 (74.2692, -80.735) -> (67.9993, -80.735)
  line L22 (67.9993, -80.735) -> (67.9993, -79.0099)
  line L23 (67.9993, -79.0099) -> (67.0197, -79.0099)
  line L24 (67.0197, -79.0099) -> (67.0197, -75.7107)
  line L25 (67.0197, -75.7107) -> (67.9993, -75.7107)
  line L26 (67.9993, -75.7107) -> (67.9993, -73.9856)
  line L27 (67.9993, -73.9856) -> (72.4697, -73.9856)
  line L28 (72.4697, -73.9856) -> (72.4697, -72.4598)
  line L29 (72.4697, -72.4598) -> (67.7693, -72.4598)
  line L30 (67.7693, -72.4598) -> (67.7693, -58.4606)
  line L31 (67.7693, -58.4606) -> (72.4697, -58.4606)
  line L32 (72.4697, -58.4606) -> (72.4697, -56.9352)
  line L33 (72.4697, -56.9352) -> (67.9993, -56.9352)
  line L34 (67.9993, -56.9352) -> (67.9993, -55.2097)
  line L35 (67.9993, -55.2097) -> (67.0197, -55.2097)
  line L36 (67.0197, -55.2097) -> (67.0197, -51.9105)
  line L37 (67.0197, -51.9105) -> (67.9993, -51.9105)
  line L38 (67.9993, -51.9105) -> (67.9993, -50.1855)
  line L39 (67.9993, -50.1855) -> (74.2692, -50.1855)
  line L40 (74.2692, -50.1855) -> (74.2692, -49.36)
  line L41 (74.2692, -49.36) -> (77.0696, -49.36)
  line L42 (77.0696, -49.36) -> (77.0696, -50.1855)
  line L43 (77.0696, -50.1855) -> (80.2996, -50.1855)
  line L44 (80.2996, -50.1855) -> (80.2996, -51.9105)
  line L45 (80.2996, -51.9105) -> (81.219, -51.9105)
  line L46 (81.219, -51.9105) -> (81.219, -55.2097)
  line L47 (81.219, -55.2097) -> (80.2996, -55.2097)
  line L48 (80.2996, -55.2097) -> (80.2996, -56.9352)
  line L49 (80.2996, -56.9352) -> (77.0696, -56.9352)
  line L50 (77.0696, -56.9352) -> (77.0696, -58.4606)
  line L51 (77.0696, -58.4606) -> (81.77, -58.4606)
  line L52 (24.62, -87.0356) -> (24.62, -101.035)
  line L53 (24.62, -101.035) -> (10.6192, -101.035)
  line L54 (10.6192, -101.035) -> (10.6192, -87.0356)
  line L55 (10.6192, -87.0356) -> (24.62, -87.0356)
  line L56 (60.9446, -129.035) -> (31.4446, -129.035)
  line L57 (31.4446, -129.035) -> (31.4446, -114.035)
  line L58 (31.4446, -114.035) -> (60.9446, -114.035)
  line L59 (60.9446, -114.035) -> (60.9446, -129.035)
  line L60 (67.7693, -87.0356) -> (81.77, -87.0356)
  line L61 (81.77, -87.0356) -> (81.77, -101.035)
  line L62 (81.77, -101.035) -> (67.7693, -101.035)
  line L63 (67.7693, -101.035) -> (67.7693, -87.0356)
  line L64 (48.7193, -67.9856) -> (62.72, -67.9856)
  line L65 (62.72, -67.9856) -> (62.72, -81.9848)
  line L66 (62.72, -81.9848) -> (48.7193, -81.9848)
  line L67 (48.7193, -81.9848) -> (48.7193, -67.9856)
  line L68 (29.6692, -81.9848) -> (29.6692, -67.9856)
  line L69 (29.6692, -67.9856) -> (43.67, -67.9856)
  line L70 (43.67, -67.9856) -> (43.67, -81.9848)
  line L71 (43.67, -81.9848) -> (29.6692, -81.9848)
  line L72 (29.6692, -62.9348) -> (29.6692, -48.9356)
  line L73 (29.6692, -48.9356) -> (43.67, -48.9356)
  line L74 (43.67, -48.9356) -> (43.67, -62.9348)
  line L75 (43.67, -62.9348) -> (29.6692, -62.9348)
  line L76 (67.9993, -13.8107) -> (67.9993, -12.0854)
  line L77 (67.9993, -12.0854) -> (74.2692, -12.0854)
  line L78 (74.2692, -12.0854) -> (74.2692, -11.26)
  line L79 (74.2692, -11.26) -> (77.0696, -11.26)
  line L80 (77.0696, -11.26) -> (77.0696, -12.0854)
  line L81 (77.0696, -12.0854) -> (80.2996, -12.0854)
  line L82 (80.2996, -12.0854) -> (80.2996, -13.8107)
  line L83 (80.2996, -13.8107) -> (81.219, -13.8107)
  line L84 (81.219, -13.8107) -> (81.219, -17.1097)
  line L85 (81.219, -17.1097) -> (80.2996, -17.1097)
  line L86 (80.2996, -17.1097) -> (80.2996, -18.835)
  line L87 (80.2996, -18.835) -> (77.0696, -18.835)
  line L88 (77.0696, -18.835) -> (77.0696, -20.3605)
  line L89 (77.0696, -20.3605) -> (81.77, -20.3605)
  line L90 (81.77, -20.3605) -> (81.77, -34.36)
  line L91 (81.77, -34.36) -> (77.0696, -34.36)
  line L92 (77.0696, -34.36) -> (77.0696, -35.8856)
  line L93 (77.0696, -35.8856) -> (80.2996, -35.8856)
  line L94 (80.2996, -35.8856) -> (80.2996, -37.6107)
  line L95 (80.2996, -37.6107) -> (81.219, -37.6107)
  line L96 (81.219, -37.6107) -> (81.219, -40.9099)
  line L97 (81.219, -40.9099) -> (80.2996, -40.9099)
  line L98 (80.2996, -40.9099) -> (80.2996, -42.635)
  line L99 (80.2996, -42.635) -> (77.0696, -42.635)
  line L100 (77.0696, -42.635) -> (77.0696, -43.4605)
  line L101 (77.0696, -43.4605) -> (74.2692, -43.4605)
  line L102 (74.2692, -43.4605) -> (74.2692, -42.635)
  line L103 (74.2692, -42.635) -> (67.9993, -42.635)
  line L104 (67.9993, -42.635) -> (67.9993, -40.9099)
  line L105 (67.9993, -40.9099) -> (67.0197, -40.9099)
  line L106 (67.0197, -40.9099) -> (67.0197, -37.6107)
  line L107 (67.0197, -37.6107) -> (67.9993, -37.6107)
  line L108 (67.9993, -37.6107) -> (67.9993, -35.8856)
  line L109 (67.9993, -35.8856) -> (72.4697, -35.8856)
  line L110 (72.4697, -35.8856) -> (72.4697, -34.36)
  line L111 (72.4697, -34.36) -> (67.7693, -34.36)
  line L112 (67.7693, -34.36) -> (67.7693, -20.3605)
  line L113 (67.7693, -20.3605) -> (72.4697, -20.3605)
  line L114 (72.4697, -20.3605) -> (72.4697, -18.835)
  line L115 (72.4697, -18.835) -> (67.9993, -18.835)
  line L116 (67.9993, -18.835) -> (67.9993, -17.1097)
  line L117 (67.9993, -17.1097) -> (67.0197, -17.1097)
  line L118 (67.0197, -17.1097) -> (67.0197, -13.8107)
  line L119 (67.0197, -13.8107) -> (67.9993, -13.8107)
  line L120 (29.6692, -43.8849) -> (29.6692, -29.8855)
  line L121 (29.6692, -29.8855) -> (43.67, -29.8855)
  line L122 (43.67, -29.8855) -> (43.67, -43.8849)
  line L123 (43.67, -43.8849) -> (29.6692, -43.8849)
  line L124 (62.72, -62.9348) -> (48.7193, -62.9348)
  line L125 (48.7193, -62.9348) -> (48.7193, -48.9356)
  line L126 (48.7193, -48.9356) -> (62.72, -48.9356)
  line L127 (62.72, -48.9356) -> (62.72, -62.9348)
  line L128 (24.62, -29.8855) -> (24.62, -43.8849)
  line L129 (24.62, -43.8849) -> (10.6192, -43.8849)
  line L130 (10.6192, -43.8849) -> (10.6192, -29.8855)
  line L131 (10.6192, -29.8855) -> (24.62, -29.8855)
  line L132 (48.7193, -24.835) -> (48.7193, -10.8355)
  line L133 (48.7193, -10.8355) -> (62.72, -10.8355)
  line L134 (62.72, -10.8355) -> (62.72, -24.835)
  line L135 (62.72, -24.835) -> (48.7193, -24.835)
  line L136 (37.3944, -24.2852) -> (37.3944, -23.3646)
  line L137 (37.3944, -23.3646) -> (35.669, -23.3646)
  line L138 (35.669, -23.3646) -> (35.669, -20.1345)
  line L139 (35.669, -20.1345) -> (34.145, -20.1345)
  line L140 (34.145, -20.1345) -> (34.145, -24.835)
  line L141 (34.145, -24.835) -> (20.1442, -24.835)
  line L142 (20.1442, -24.835) -> (20.1442, -20.1345)
  line L143 (20.1442, -20.1345) -> (18.6201, -20.1345)
  line L144 (18.6201, -20.1345) -> (18.6201, -23.3646)
  line L145 (18.6201, -23.3646) -> (16.8934, -23.3646)
  line L146 (16.8934, -23.3646) -> (16.8934, -24.2852)
  line L147 (16.8934, -24.2852) -> (13.593, -24.2852)
  line L148 (13.593, -24.2852) -> (13.593, -23.3646)
  line L149 (13.593, -23.3646) -> (11.869, -23.3646)
  line L150 (11.869, -23.3646) -> (11.869, -20.1345)
  line L151 (11.869, -20.1345) -> (11.0436, -20.1345)
  line L152 (11.0436, -20.1345) -> (11.0436, -17.3357)
  line L153 (11.0436, -17.3357) -> (11.869, -17.3357)
  line L154 (11.869, -17.3357) -> (11.869, -11.0657)
  line L155 (11.869, -11.0657) -> (13.593, -11.0657)
  line L156 (13.593, -11.0657) -> (13.593, -10.0858)
  line L157 (13.593, -10.0858) -> (16.8934, -10.0858)
  line L158 (16.8934, -10.0858) -> (16.8934, -11.0657)
  line L159 (16.8934, -11.0657) -> (18.6201, -11.0657)
  line L160 (18.6201, -11.0657) -> (18.6201, -15.5346)
  line L161 (18.6201, -15.5346) -> (20.1442, -15.5346)
  line L162 (20.1442, -15.5346) -> (20.1442, -10.8355)
  line L163 (20.1442, -10.8355) -> (34.145, -10.8355)
  line L164 (34.145, -10.8355) -> (34.145, -15.5346)
  line L165 (34.145, -15.5346) -> (35.669, -15.5346)
  line L166 (35.669, -15.5346) -> (35.669, -11.0657)
  line L167 (35.669, -11.0657) -> (37.3944, -11.0657)
  line L168 (37.3944, -11.0657) -> (37.3944, -10.0858)
  line L169 (37.3944, -10.0858) -> (40.6936, -10.0858)
  line L170 (40.6936, -10.0858) -> (40.6936, -11.0657)
  line L171 (40.6936, -11.0657) -> (42.4187, -11.0657)
  line L172 (42.4187, -11.0657) -> (42.4187, -17.3357)
  line L173 (42.4187, -17.3357) -> (43.2442, -17.3357)
  line L174 (43.2442, -17.3357) -> (43.2442, -20.1345)
  line L175 (43.2442, -20.1345) -> (42.4187, -20.1345)
  line L176 (42.4187, -20.1345) -> (42.4187, -23.3646)
  line L177 (42.4187, -23.3646) -> (40.6936, -23.3646)
  line L178 (40.6936, -23.3646) -> (40.6936, -24.2852)
  line L179 (40.6936, -24.2852) -> (37.3944, -24.2852)
  line L180 (62.72, -29.8855) -> (62.72, -43.8849)
  line L181 (62.72, -43.8849) -> (48.7193, -43.8849)
  line L182 (48.7193, -43.8849) -> (48.7193, -29.8855)
  line L183 (48.7193, -29.8855) -> (62.72, -29.8855)
  line L184 (29.6692, -87.0356) -> (43.67, -87.0356)
  line L185 (43.67, -87.0356) -> (43.67, -101.035)
  line L186 (43.67, -101.035) -> (29.6692, -101.035)
  line L187 (29.6692, -101.035) -> (29.6692, -87.0356)
  line L188 (24.62, -48.9356) -> (24.62, -62.9348)
  line L189 (24.62, -62.9348) -> (10.6192, -62.9348)
  line L190 (10.6192, -62.9348) -> (10.6192, -48.9356)
  line L191 (10.6192, -48.9356) -> (24.62, -48.9356)
  arc A2 (4.6192, -140.035) -> (6.6192, -142.035) centre (6.6192, -140.035) ccw
  line L192 (6.6192, -142.035) -> (85.77, -142.035)
  arc A3 (85.77, -142.035) -> (87.77, -140.035) centre (85.77, -140.035) ccw
  line L193 (87.77, -140.035) -> (87.77, -6.8355)
  arc A4 (87.77, -6.8355) -> (85.77, -4.8355) centre (85.77, -6.8355) ccw
  line L194 (85.77, -4.8355) -> (6.6192, -4.8355)
  arc A5 (6.6192, -4.8355) -> (4.6192, -6.8355) centre (6.6192, -6.8355) ccw
  line L195 (4.6192, -6.8355) -> (4.6192, -140.035)
  line L196 (20.1442, -10.8355) -> (10.6192, -10.8355) construction
  line L197 (10.6192, -10.8355) -> (10.6192, -29.8855) construction
  line L198 (5.205, -5.4213) -> (10.6192, -10.8355) construction
  circle A6 centre (6.9121, -7.1284) radius 1
  line L199 (10.6192, -128.5347) -> (10.6192, -114.5353)
  line L200 (10.6192, -114.5353) -> (24.62, -114.5353)
  line L201 (24.62, -114.5353) -> (24.62, -128.5347)
  line L202 (24.62, -128.5347) -> (10.6192, -128.5347)
  dimension "d130" = 2
  constraint coincident L162.end L163.start
  constraint perpendicular L130 L196
  constraint coincident L130.end L131.start
  constraint perpendicular L131 L197
  constraint midpoint A5 L198.start
  constraint coincident L198 A6.centre
  measures "d130" diameter of A6
extrude "Extrude3'" cut sketch "Sketch7" against normal up to surface (4.9 mm away) contours A6 bodies 1 in component "Plate"
extrude "Extrude7" cut sketch "Sketch7" against normal up to surface (4.9 mm away) contours A6 bodies 2 in component "Top"
mirror "Mirror2" about plane through (46.1946, 73.4353, 1.075) normal (-1, 0, 0) of "Extrude3'" in component "Plate"
mirror "Mirror2'" about plane through (46.1946, 73.4353, 1.075) normal (-1, 0, 0) of "Extrude7" in component "Top"
sketch "Sketch5 (2)" plane through (0, 0, 8.15) normal (0, 0, 1) x (-1, 0, 0) in component "Top"
  arc A0 (-95.92, -148.185) -> (-93.92, -150.185) centre (-93.92, -148.185) ccw
  line L0 (-93.92, -150.185) -> (1.5308, -150.185)
  arc A1 (1.5308, -150.185) -> (3.5308, -148.185) centre (1.5308, -148.185) ccw
  line L1 (3.5308, -148.185) -> (3.5308, 1.3145)
  arc A2 (3.5308, 1.3145) -> (1.5308, 3.3145) centre (1.5308, 1.3145) ccw
  line L2 (1.5308, 3.3145) -> (-93.92, 3.3145)
  arc A3 (-93.92, 3.3145) -> (-95.92, 1.3145) centre (-93.92, 1.3145) ccw
  line L3 (-95.92, 1.3145) -> (-95.92, -148.185)
  line L4 (-83.2947, -8.3103) -> (-9.0946, -8.3102)
  arc A4 (-8.0946, -9.3102) -> (-9.0946, -8.3102) centre (-9.0946, -9.3102) ccw
  line L5 (-8.0946, -9.3102) -> (-8.0946, -102.5603)
  arc A5 (-9.0946, -103.5603) -> (-8.0946, -102.5603) centre (-9.0946, -102.5603) ccw
  line L6 (-9.0946, -103.5603) -> (-83.2947, -103.5603)
  arc A6 (-84.2947, -102.5603) -> (-83.2947, -103.5603) centre (-83.2947, -102.5603) ccw
  line L7 (-84.2947, -102.5603) -> (-84.2947, -9.3102)
  arc A7 (-83.2947, -8.3102) -> (-84.2947, -9.3102) centre (-83.2947, -9.3103) ccw
sketch "Sketch6 (2)" plane through (0, 0, 8.15) normal (0, 0, 1) x (-1, 0, 0) in component "Top"
  arc A0 (-95.92, -148.185) -> (-93.92, -150.185) centre (-93.92, -148.185) ccw
  line L0 (-93.92, -150.185) -> (1.5308, -150.185)
  arc A1 (1.5308, -150.185) -> (3.5308, -148.185) centre (1.5308, -148.185) ccw
  line L1 (3.5308, -148.185) -> (3.5308, 1.3145)
  arc A2 (3.5308, 1.3145) -> (1.5308, 3.3145) centre (1.5308, 1.3145) ccw
  line L2 (1.5308, 3.3145) -> (-93.92, 3.3145)
  arc A3 (-93.92, 3.3145) -> (-95.92, 1.3145) centre (-93.92, 1.3145) ccw
  line L3 (-95.92, 1.3145) -> (-95.92, -148.185)
  line L4 (-83.2947, -8.3103) -> (-9.0946, -8.3102)
  arc A4 (-8.0946, -9.3102) -> (-9.0946, -8.3102) centre (-9.0946, -9.3102) ccw
  line L5 (-8.0946, -9.3102) -> (-8.0946, -102.5603)
  arc A5 (-9.0946, -103.5603) -> (-8.0946, -102.5603) centre (-9.0946, -102.5603) ccw
  line L6 (-9.0946, -103.5603) -> (-83.2947, -103.5603)
  arc A6 (-84.2947, -102.5603) -> (-83.2947, -103.5603) centre (-83.2947, -102.5603) ccw
  line L7 (-84.2947, -102.5603) -> (-84.2947, -9.3102)
  arc A7 (-83.2947, -8.3102) -> (-84.2947, -9.3102) centre (-83.2947, -9.3103) ccw
sketch "Sketch7 (2)" plane through (0, 142.185, 0) normal (0, 1, 0) x (-1, 0, 0) in component "Top"